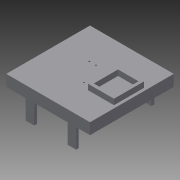
# Autodesk Inventor part: Body
Saved by Autodesk Inventor 2015 (Build 190159000, 159)
## iProperties
Created: 2015-06-13
Part Number: Body
Material: Generic
Document SubType Name: Modeling
Designer: Abhishyant
Density: 1 g/cm^3
Appearance: Default
Author: Abhishyant
Autodesk Inventor part; units mm, degrees
ref_plane "YZ Plane" through (0, 0, 0) normal (1, 0, 0) x (0, 1, 0)
ref_plane "XZ Plane" through (0, 0, 0) normal (0, 1, 0) x (-1, 0, 0)
ref_plane "XY Plane" through (0, 0, 0) normal (0, 0, 1) x (1, 0, 0)
sketch "Sketch1" plane through (0, 0, 0) normal (0, 1, 0) x (-1, 0, 0)
  line L0 (-150, -150) -> (150, -150)
  line L1 (150, -150) -> (150, 150)
  line L2 (150, 150) -> (-150, 150)
  line L3 (-150, 150) -> (-150, -150)
  line L4 (-150, -150) -> (150, 150) construction
  line L5 (150, -150) -> (-150, 150) construction
  point P0 (0, 0)
  constraints: 12 end point, 2 midpoint, 2 parallel, 1 horizontal, 1 perpendicular
extrude "Extrusion1" add sketch "Sketch1" along normal blind 40
sketch "Sketch4" plane through (0, 0, 0) normal (0, -1, 0) x (1, 0, 0)
  line L0 (150, -150) -> (-150, -150) projected
  line L1 (0, -150) -> (150, -150)
  line L2 (60, -130) -> (90, -130)
  line L3 (90, -130) -> (90, -140)
  line L4 (90, -140) -> (60, -140)
  line L5 (60, -140) -> (60, -130)
  line L6 (60, -130) -> (90, -140) construction
  line L7 (90, -130) -> (60, -140) construction
  line L8 (-60, -130) -> (-90, -130)
  line L9 (-90, -130) -> (-90, -140)
  line L10 (-90, -140) -> (-60, -140)
  line L11 (-60, -140) -> (-60, -130)
  line L12 (150, 150) -> (150, -150) projected
  line L13 (60, 130) -> (90, 130)
  line L14 (90, 130) -> (90, 140)
  line L15 (90, 140) -> (60, 140)
  line L16 (60, 140) -> (60, 130)
  line L17 (60, 130) -> (90, 140) construction
  line L18 (90, 130) -> (60, 140) construction
  line L19 (-60, 130) -> (-90, 130)
  line L20 (-60, 140) -> (-60, 130)
  line L21 (-90, 140) -> (-60, 140)
  line L22 (-90, 130) -> (-90, 140)
  point P0 (0, 0)
  constraints: 42 end point, 2 parallel, 1 collinear, 1 horizontal, 1 midpoint, 1 perpendicular
extrude "Extrusion3" add sketch "Sketch4" along normal blind 30
sketch "Sketch5" plane through (0, 0, 0) normal (0, -1, 0) x (1, 0, 0)
  line L0 (-40, 22.5) -> (-50, 22.5)
  line L1 (-50, 22.5) -> (-50, -22.5)
  line L2 (-50, -22.5) -> (-40, -22.5)
  line L3 (-40, -22.5) -> (-40, 22.5)
  line L4 (-40, 22.5) -> (-50, -22.5) construction
  line L5 (-50, 22.5) -> (-40, -22.5) construction
  line L6 (-16, -22.5) -> (-6, -22.5)
  line L7 (-6, -22.5) -> (-6, 22.5)
  line L8 (-6, 22.5) -> (-16, 22.5)
  line L9 (-16, 22.5) -> (-16, -22.5)
  line L10 (40, 22.5) -> (50, 22.5)
  line L11 (50, 22.5) -> (50, -22.5)
  line L12 (50, -22.5) -> (40, -22.5)
  line L13 (40, -22.5) -> (40, 22.5)
  line L14 (40, 22.5) -> (50, -22.5) construction
  line L15 (50, 22.5) -> (40, -22.5) construction
  line L16 (16, -22.5) -> (6, -22.5)
  line L17 (6, -22.5) -> (6, 22.5)
  line L18 (6, 22.5) -> (16, 22.5)
  line L19 (16, 22.5) -> (16, -22.5)
  point P0 (0, 0)
  point P1 (-45, 0)
  point P2 (45, 0)
  constraints: 40 end point, 4 midpoint, 4 parallel, 2 horizontal, 2 perpendicular
extrude "Extrusion4" add sketch "Sketch5" along normal blind 30
sketch "Sketch6" plane through (40, 0, -22.5) normal (-1, 0, 0) x (0, 0, 1)
  line L0 (0, 0) -> (0, -30) projected
  line L1 (45, -30) -> (0, -30)
  line L2 (0, -30) -> (0, -24)
  line L3 (0, -24) -> (45, -24)
  line L4 (45, -24) -> (45, -30)
  point P0 (22.5, 0)
  constraints: 8 end point, 2 parallel, 1 horizontal, 1 perpendicular, 1 point on line
extrude "Extrusion5" add sketch "Sketch6" along normal blind 24
sketch "Sketch9" plane through (-40, 0, 22.5) normal (1, 0, 0) x (0, 0, -1)
  line L0 (0, 0) -> (0, -30) projected
  line L1 (45, -30) -> (0, -30)
  line L2 (0, -30) -> (0, -24)
  line L3 (0, -24) -> (45, -24)
  line L4 (45, -24) -> (45, -30)
  point P0 (22.5, 0)
  constraints: 8 end point, 2 parallel, 1 horizontal, 1 perpendicular, 1 point on line
extrude "Extrusion6" add sketch "Sketch9" along normal blind 24
sketch "Sketch12" plane through (0, 0, 0) normal (0, -1, 0) x (1, 0, 0)
  circle A0 centre (-40, -37.5) radius 2.5
  circle A1 centre (-16, -37.5) radius 2.5
  line L0 (0, 0) -> (11, 0)
  circle A2 centre (16, 37.5) radius 2.5
  circle A3 centre (40, 37.5) radius 2.5
  constraints: 4 centre point, 2 end point, 1 horizontal
hole "Hole1" at (-40, 0, -37.5) at (-16, 0, -37.5) at (16, 0, 37.5) at (40, 0, 37.5) direction (0, 1, 0) diameter 5 end through all
sketch "Sketch14" plane through (0, 40, 0) normal (0, 1, 0) x (1, 0, 0)
  line L0 (150, -150) -> (150, 150) projected
  line L1 (150, 0) -> (150, 34.3)
  line L2 (130, 33.8503) -> (130, 43.8503)
  line L3 (130, 43.8503) -> (56.6, 43.8503)
  line L4 (56.6, 43.8503) -> (56.6, -42.9497)
  line L5 (56.6, -42.9497) -> (130, -42.9497)
  line L6 (130, -42.9497) -> (130, 43.8503)
  line L7 (66.6, 43.8503) -> (56.6, 43.8503)
  line L8 (130, 53.8503) -> (140, 53.8503)
  line L9 (140, 53.8503) -> (46.6, 53.8503)
  line L10 (46.6, 53.8503) -> (46.6, -54.1497)
  line L11 (46.6, -54.1497) -> (140, -54.1497)
  line L12 (140, -54.1497) -> (140, 53.8503)
  point P0 (0, 0)
  constraints: 24 end point, 4 parallel, 3 horizontal, 2 perpendicular, 1 midpoint, 1 point on line, 1 vertical
extrude "Extrusion10" add sketch "Sketch14" along normal blind 20
sketch "Sketch17" plane through (0, -30, 0) normal (0, -1, 0) x (1, 0, 0)
  line L0 (-90, 130) -> (-60, 130) projected
  line L1 (-60, 130) -> (-60, 140) projected
  line L2 (-60, 140) -> (-90, 140) projected
  line L3 (-90, 140) -> (-90, 130) projected
  point P0 (0, 0)
sketch "Sketch18" plane through (0, -30, 0) normal (0, -1, 0) x (1, 0, 0)
  line L0 (60, 130) -> (90, 130) projected
  line L1 (90, 130) -> (90, 140) projected
  line L2 (90, 140) -> (60, 140) projected
  line L3 (60, 140) -> (60, 130) projected
  point P0 (0, 0)
sketch "Sketch19" plane through (0, -30, 0) normal (0, -1, 0) x (1, 0, 0)
  line L0 (-60, -130) -> (-90, -130) projected
  line L1 (-90, -130) -> (-90, -140) projected
  line L2 (-90, -140) -> (-60, -140) projected
  line L3 (-60, -140) -> (-60, -130) projected
  point P0 (0, 0)
sketch "Sketch20" plane through (0, -30, 0) normal (0, -1, 0) x (1, 0, 0)
  line L0 (90, -130) -> (60, -130) projected
  line L1 (60, -130) -> (60, -140) projected
  line L2 (60, -140) -> (90, -140) projected
  line L3 (90, -140) -> (90, -130) projected
  point P0 (0, 0)
extrude "Extrusion11" add sketch "Sketch17" along normal blind 50
extrude "Extrusion12" add sketch "Sketch19" along normal blind 50
extrude "Extrusion13" add sketch "Sketch20" along normal blind 50
extrude "Extrusion14" add sketch "Sketch18" along normal blind 50
body "Solid1"
